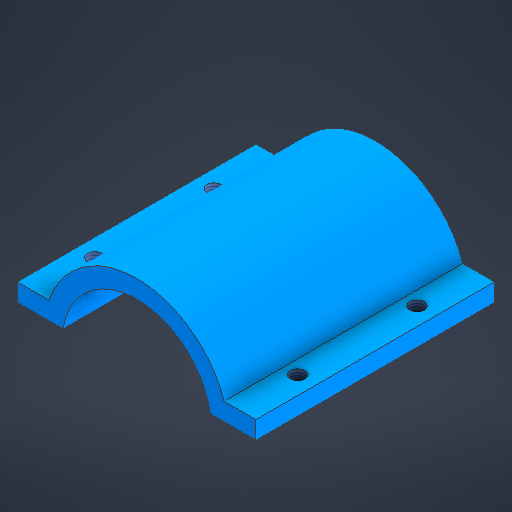
# Autodesk Inventor part: Part2
Saved by Autodesk Inventor 2026.1 (Build 301233000, 233)
## iProperties
Created: 2025-08-21
Part Number: Part2
Material: Generic
Document SubType Name: Modeling
Designer: ASUS
Density: 1 g/cm^3
Appearance: Default
Author: ASUS
Autodesk Inventor part; units mm, degrees
ref_plane "YZ Plane" through (0, 0, 0) normal (1, 0, 0) x (0, 1, 0)
ref_plane "XZ Plane" through (0, 0, 0) normal (0, 1, 0) x (-1, 0, 0)
ref_plane "XY Plane" through (0, 0, 0) normal (0, 0, 1) x (1, 0, 0)
sketch "Sketch1" plane through (0, 0, 0) normal (0, 0, 1) x (1, 0, 0)
  line L0 (0, 0) -> (0, 3)
  arc A0 (32.339, 0) -> (7.661, 0) centre (20, -2) ccw
  line L1 (0, 0) -> (7.661, 0)
  arc A1 (34.2916, 4) -> (5.3286, 3) centre (20, -2) ccw
  line L2 (0, 3) -> (5.3286, 3)
  line L3 (40, 0) -> (40, 3)
  line L4 (32.339, 0) -> (40, 0)
  line L5 (20, -2) -> (20, 11.991)
  line L6 (40, 0) -> (40, 3)
  line L7 (40, 0) -> (32.339, 0)
  arc A2 (34.6714, 3) -> (5.7084, 4) centre (20, -2) ccw
  line L8 (40, 3) -> (34.6714, 3)
  dimension "d12" = 20
  dimension "d14" = 25
  dimension "d38" = 2
  dimension "d40" = 3
  dimension "d41" = 40
  dimension "d57" = 3
  constraints: 18 end point, 6 point on circle, 3 centre point, 2 horizontal, 2 symmetric about line, 2 vertical, 1 parallel, 1 perpendicular, 1 other
  measures "d12" horizontal distance of L0.start L5.start
  measures "d14" diameter of A0
  measures "d38" vertical distance of L0.start L5.start
  measures "d40" distance of L3.start L3.end
  measures "d41" distance of L0.start L3.start
  measures "d57" radial gap between concentric circles of A0 A1
extrude "Extrusion1" add sketch "Sketch1" along normal blind 40
sketch "Sketch3" plane through (0, 3, 0) normal (0, 1, 0) x (1, 0, 0)
  line L0 (5.3286, 0) -> (0, 0) projected
  line L1 (5.3286, -40) -> (0, -40) projected
  line L2 (0, 0) -> (0, -40) projected
  line L3 (40, 0) -> (40, -40) projected
  point P0 (3, -10)
  point P1 (3, -30)
  point P2 (37, -10)
  point P3 (37, -30)
  dimension "d42" = 10
  dimension "d43" = 20
  dimension "d45" = 20
  dimension "d53" = 3
  dimension "d54" = 3
  dimension "d55" = 3
  dimension "d56" = 3
  measures "d42" distance from line of L0 point (3, -10)
  measures "d43" distance of point (3, -30) point (3, -10)
  measures "d45" distance of point (37, -10) point (37, -30)
  measures "d53" distance from line of L2 point (3, -10)
  measures "d54" distance from line of L2 point (3, -30)
  measures "d55" distance from line of L3 point (37, -10)
  measures "d56" distance from line of L3 point (37, -30)
hole "Hole2" at (3, 3, 10) at (3, 3, 30) at (37, 3, 10) at (37, 3, 30) direction (0, -1, 0) diameter 2.459 end through all thread size "M3x0.5" class "6H" standard "ISO Metric profile"
body "Solid1"
